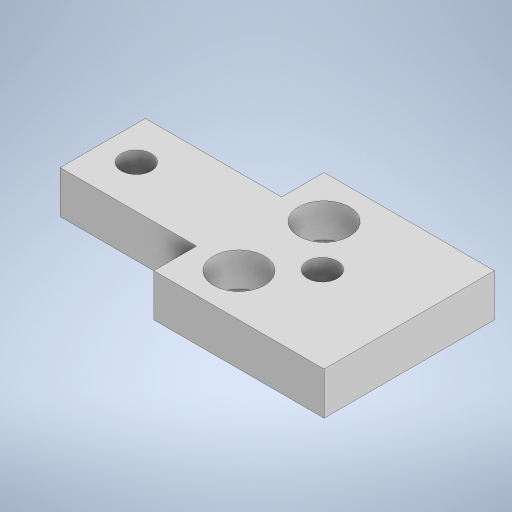
# Autodesk Inventor part: DovetailSampleHolderToKB1X1TMagneticHolder
Saved by Autodesk Inventor 2024.2 (Build 282272000, 272)
## iProperties
Created: 2024-12-11
Part Number: DovetailSampleHolderToKB1X1TMagneticHolder
Material: Generic
Document SubType Name: Modeling
Designer: monolithic
Density: 1 g/cm^3
Appearance: Default
Author: monolithic
Autodesk Inventor part; units mm, degrees
ref_plane "YZ Plane" through (0, 0, 0) normal (1, 0, 0) x (0, 1, 0)
ref_plane "XZ Plane" through (0, 0, 0) normal (0, 1, 0) x (-1, 0, 0)
ref_plane "XY Plane" through (0, 0, 0) normal (0, 0, 1) x (1, 0, 0)
sketch "Sketch1" plane through (0, 0, 0) normal (0, 1, 0) x (-1, 0, 0)
  line L0 (0, 0) -> (-25.4, 0)
  line L1 (-25.4, 0) -> (-25.4, -25.4)
  line L2 (-25.4, -25.4) -> (0, -25.4)
  line L3 (0, -25.4) -> (0, 0)
  line L4 (0, 0) -> (0, -6.35)
  line L5 (0, -6.35) -> (-6.35, -6.35)
  line L6 (-6.35, -6.35) -> (-6.35, -19.05)
  line L7 (0, -12.7) -> (-12.446, -12.7)
  circle A0 centre (-6.35, -6.35) radius 2.25
  circle A1 centre (-6.35, -19.05) radius 2.25
  circle A2 centre (-12.7, -12.7) radius 2.25
  circle A3 centre (-12.446, -12.7) radius 2.25
  dimension "d0" = 25.4
  dimension "d1" = 25.4
  dimension "d2" = 6.35
  dimension "d3" = 6.35
  dimension "d4" = 12.7
  dimension "d5" = 12.446
  dimension "d6" = 4.5
  dimension "d7" = 4.5
  dimension "d8" = 4.5
  dimension "d20" = 4.5
  constraints: 16 end point, 4 centre point, 3 coincident, 3 perpendicular, 2 horizontal, 2 parallel, 1 midpoint, 1 point on line
  measures "d0" distance of L0.end L1.end
  measures "d1" distance of L1.end L2.end
  measures "d2" distance of L0.start L4.end
  measures "d3" distance of L4.end L5.end
  measures "d4" distance of L5.end L6.end
  measures "d5" distance of L7.start L7.end
  measures "d6" diameter of A0
  measures "d7" diameter of A1
  measures "d8" diameter of A2
  measures "d20" diameter of A3
extrude "Extrusion1" add sketch "Sketch1" along normal blind 6.35 contours L3 L5 A0 L6 L7 L2 L1 L0 | L3 L7 L6 A0 L5 | A3 A2 picked at (-14.7705, -12.7)
sketch "Sketch2" plane through (0, 6.35, 0) normal (0, 1, 0) x (1, 0, 0)
  circle A0 centre (12.7, 12.7) radius 2.25 projected
  line L0 (0, 25.4) -> (0, 0) projected
  line L1 (0, 0) -> (25.4, 0) projected
  line L2 (25.4, 0) -> (25.4, 25.4) projected
  line L3 (25.4, 25.4) -> (0, 25.4) projected
  line L4 (0, 25.4) -> (0, 0) projected
  circle A1 centre (6.35, 19.05) radius 2.25 projected
  circle A2 centre (6.35, 6.35) radius 2.25 projected
  line L5 (12.7, 12.7) -> (-15.325, 12.7)
  circle A3 centre (-15.325, 12.7) radius 2.25
  line L6 (0, 19.05) -> (-20.32, 19.05)
  line L7 (-20.32, 19.05) -> (-20.32, 6.35)
  line L8 (-20.32, 6.35) -> (0, 6.35)
  line L9 (0, 6.35) -> (0, 19.05)
  point P0 (0, 6.35)
  dimension "d11" = 28.025
  dimension "d12" = 4.5
  dimension "d13" = 20.32
  constraints: 10 end point, 2 horizontal, 2 parallel, 1 centre point, 1 coincident, 1 perpendicular, 1 point on line
  measures "d11" distance of L5.start L5.end
  measures "d12" diameter of A3
  measures "d13" distance of L8.end L7.end
extrude "Extrusion2" add sketch "Sketch2" against normal blind 6.35 contours L0 L8 L7 L6
sketch "Sketch3" plane through (0, 6.35, 0) normal (0, 1, 0) x (1, 0, 0)
  circle A0 centre (12.7, 12.7) radius 2.25 projected
  circle A1 centre (6.35, 19.05) radius 2.25 projected
  circle A2 centre (6.35, 6.35) radius 2.25 projected
  circle A3 centre (6.35, 19.05) radius 3.81
  circle A4 centre (6.35, 6.35) radius 3.81
  point P0 (0, 0)
  dimension "d16" = 7.62
  dimension "d17" = 7.62
  constraints: 2 centre point, 2 coincident
  measures "d16" diameter of A3
  measures "d17" diameter of A4
extrude "Extrusion3" cut sketch "Sketch3" against normal blind 5.08 contours A1 | A2 | A3 | A4
body "Solid1"
